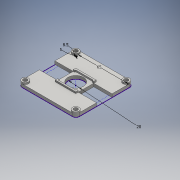
# Autodesk Inventor part: 20mm glass cuvette holder
Saved by Autodesk Inventor 2016 SP1 (Build 200210100, 210)
## iProperties
Created: 2015-08-25
Part Number: 20mm glass cuvette holder
Material: Generic
Document SubType Name: Modeling
Designer: kthorn
Density: 1 g/cm^3
Appearance: Default
Author: kthorn
Autodesk Inventor part; units mm, degrees
ref_plane "YZ Plane" through (0, 0, 0) normal (1, 0, 0) x (0, 1, 0)
ref_plane "XZ Plane" through (0, 0, 0) normal (0, 1, 0) x (-1, 0, 0)
ref_plane "XY Plane" through (0, 0, 0) normal (0, 0, 1) x (1, 0, 0)
sketch "Sketch1" plane through (0, 0, 0) normal (0, 0, 1) x (1, 0, 0)
  line L0 (-32.5, 32.5) -> (32.5, 32.5) construction
  line L1 (32.5, 32.5) -> (32.5, -32.5) construction
  line L2 (32.5, -32.5) -> (-32.5, -32.5) construction
  line L3 (-32.5, -32.5) -> (-32.5, 32.5) construction
  circle A0 centre (-32.5, 32.5) radius 2.5
  circle A1 centre (32.5, 32.5) radius 2.5
  circle A2 centre (-32.5, -32.5) radius 2.5
  circle A3 centre (32.5, -32.5) radius 2.5
  line L4 (-32.5, 32.5) -> (32.5, -32.5) construction
  circle A4 centre (0, 0) radius 10
  circle A5 centre (-32.5, 32.5) radius 4.25
  circle A6 centre (32.5, 32.5) radius 4.25
  circle A7 centre (-32.5, -32.5) radius 4.25
  circle A8 centre (32.5, -32.5) radius 4.25
  line L5 (-32.5, 36.75) -> (32.5, 36.75)
  line L6 (32.5, -36.75) -> (-32.5, -36.75)
  line L7 (-36.75, 32.5) -> (-36.75, -32.5)
  line L8 (36.75, 32.5) -> (36.75, -32.5)
  dimension "d1" = 65
  dimension "d2" = 5
  dimension "d4" = 20
  dimension "d16" = 8.5
  constraints: 18 end point, 9 centre point, 9 coincident, 8 point on circle, 7 tangent, 6 equal radius, 2 horizontal, 2 parallel, 2 perpendicular, 1 midpoint
  measures "d1" distance of L0.start L0.end
  measures "d2" diameter of A0
  measures "d4" diameter of A4
  measures "d16" diameter of A5
extrude "Extrusion1" add sketch "Sketch1" along normal blind 4
sketch "Sketch2" plane through (0, 0, 4) normal (0, 0, 1) x (1, 0, 0)
  line L0 (-11.2, 11.2) -> (11.2, 11.2)
  line L1 (11.2, -11.2) -> (-11.2, -11.2)
  line L2 (0, 11.2) -> (0, 36.75) construction
  line L3 (0, -11.2) -> (0, -36.75) construction
  line L4 (-13.2, 13.2) -> (13.2, 13.2)
  line L5 (13.2, -13.2) -> (-13.2, -13.2)
  line L6 (11.2, 11.2) -> (13.2, 13.2) construction
  line L7 (-11.2, 11.2) -> (-13.2, 13.2) construction
  line L8 (-13.2, -13.2) -> (-11.2, -11.2) construction
  line L9 (11.2, -11.2) -> (13.2, -13.2) construction
  circle A0 centre (0, 0) radius 10 projected
  circle A1 centre (-32.5, -32.5) radius 2.5 projected
  circle A2 centre (32.5, -32.5) radius 2.5 projected
  circle A3 centre (32.5, 32.5) radius 2.5 projected
  circle A4 centre (-32.5, 32.5) radius 2.5 projected
  arc A5 (32.5, -36.75) -> (36.75, -32.5) centre (32.5, -32.5) ccw projected
  line L10 (36.75, -32.5) -> (36.75, 32.5) projected
  arc A6 (36.75, 32.5) -> (32.5, 36.75) centre (32.5, 32.5) ccw projected
  line L11 (32.5, 36.75) -> (-32.5, 36.75) projected
  arc A7 (-32.5, 36.75) -> (-36.75, 32.5) centre (-32.5, 32.5) ccw projected
  line L12 (-36.75, 32.5) -> (-36.75, -32.5) projected
  arc A8 (-36.75, -32.5) -> (-32.5, -36.75) centre (-32.5, -32.5) ccw projected
  line L13 (-32.5, -36.75) -> (32.5, -36.75) projected
  line L14 (-32.5, -36.75) -> (32.5, -36.75) projected
  line L15 (36.75, -32.5) -> (36.75, 32.5) projected
  line L16 (32.5, 36.75) -> (-32.5, 36.75) projected
  line L17 (-13.2, 10) -> (-11.2, 10)
  line L18 (-13.2, -10) -> (-11.2, -10)
  line L19 (-13.2, -13.2) -> (-13.2, -10)
  line L20 (-13.2, 10) -> (-13.2, 13.2)
  line L21 (-11.2, -11.2) -> (-11.2, -10)
  line L22 (-11.2, 10) -> (-11.2, 11.2)
  line L23 (11.2, 10) -> (13.2, 10)
  line L24 (11.2, -10) -> (13.2, -10)
  line L25 (11.2, 11.2) -> (11.2, 10)
  line L26 (11.2, -10) -> (11.2, -11.2)
  line L27 (13.2, 13.2) -> (13.2, 10)
  line L28 (13.2, -10) -> (13.2, -13.2)
  line L29 (-11.2, 11.2) -> (0, 0) construction
  line L30 (0, 0) -> (-11.2, -11.2) construction
  line L31 (0, 0) -> (11.2, 11.2) construction
  line L32 (0, 0) -> (11.2, -11.2) construction
  dimension "d7" = 22.4
  dimension "d24" = 2
  dimension "d31" = 2
  dimension "d34" = 20
  constraints: 52 end point, 14 perpendicular, 12 equal length, 10 parallel, 4 midpoint, 2 horizontal, 2 point on line, 1 vertical
  measures "d7" distance of L0.start L0.end
  measures "d24" distance of L17.start L17.end
  measures "d31" distance between parallel lines of L0 L4
  measures "d34" distance from line of L18.end L17
extrude "Extrusion2" add sketch "Sketch2" along normal blind 2 contours L22 L17 L20 L4 L27 L23 L25 L0 | L26 L24 L28 L5 L19 L18 L21 L1
extrude "Extrusion4" add sketch "Sketch1" along normal blind 6 contours A5 | A6 | A7 | A8
sketch "Sketch4" plane through (0, 0, 4) normal (0, 0, 1) x (1, 0, 0)
  line L0 (13.2, 13.2) -> (13.2, 10) projected
  line L1 (-13.2, 13.2) -> (13.2, 13.2) projected
  arc A0 (36.75, -32.5) -> (32.5, -36.75) centre (32.5, -32.5) ccw projected
  line L2 (36.75, -32.5) -> (36.75, 32.5) projected
  arc A1 (32.5, 36.75) -> (36.75, 32.5) centre (32.5, 32.5) ccw projected
  line L3 (32.5, 36.75) -> (-32.5, 36.75) projected
  arc A2 (-36.75, 32.5) -> (-32.5, 36.75) centre (-32.5, 32.5) ccw projected
  line L4 (-36.75, 32.5) -> (-36.75, -32.5) projected
  arc A3 (-32.5, -36.75) -> (-36.75, -32.5) centre (-32.5, -32.5) ccw projected
  line L5 (-32.5, -36.75) -> (32.5, -36.75) projected
  line L6 (-13.2, 10) -> (-13.2, -10)
  line L7 (-13.2, -10) -> (-36.75, -10)
  line L8 (-36.75, -10) -> (-36.75, 10)
  line L9 (-36.75, 10) -> (-13.2, 10)
  line L10 (32.5, 36.75) -> (-32.5, 36.75) construction
  line L11 (0, 36.75) -> (0, -36.75) construction
  line L12 (13.2, 10) -> (13.2, -10)
  line L13 (13.2, -10) -> (36.75, -10)
  line L14 (36.75, -10) -> (36.75, 10)
  line L15 (36.75, 10) -> (13.2, 10)
  line L16 (-11.2, 11.2) -> (-11.2, 10) projected
  line L17 (-11.2, 10) -> (-13.2, 10) projected
  line L18 (-13.2, 10) -> (-13.2, 13.2) projected
  line L19 (13.2, 10) -> (11.2, 10) projected
  line L20 (11.2, 10) -> (11.2, 11.2) projected
  line L21 (11.2, 11.2) -> (-11.2, 11.2) projected
  line L22 (-11.2, 11.2) -> (11.2, 11.2) projected
  line L23 (11.2, 11.2) -> (11.2, 10) projected
  line L24 (11.2, 10) -> (13.2, 10) projected
  line L25 (13.2, 10) -> (13.2, 13.2) projected
  line L26 (13.2, 13.2) -> (-13.2, 13.2) projected
  line L27 (-13.2, 13.2) -> (-13.2, 10) projected
  line L28 (-13.2, 10) -> (-11.2, 10) projected
  line L29 (-11.2, 10) -> (-11.2, 11.2) projected
  line L30 (-11.2, -11.2) -> (-11.2, -10) projected
  line L31 (-13.2, -10) -> (-13.2, -13.2) projected
  line L32 (-13.2, 13.2) -> (-13.2, 10) projected
  circle A4 centre (0, 0) radius 10 projected
  line L33 (-11.2, -11.2) -> (11.2, -11.2) projected
  line L34 (11.2, -11.2) -> (11.2, -10) projected
  line L35 (11.2, -10) -> (13.2, -10) projected
  line L36 (13.2, -10) -> (13.2, -13.2) projected
  line L37 (13.2, -13.2) -> (-13.2, -13.2) projected
  line L38 (-13.2, -13.2) -> (-13.2, -10) projected
  line L39 (-13.2, -10) -> (-11.2, -10) projected
  line L40 (-11.2, -10) -> (-11.2, -11.2) projected
  point P0 (-36.75, 0)
  point P1 (36.75, 0)
  dimension "d20" = 20
  constraints: 18 end point, 5 symmetric about line, 4 midpoint, 2 parallel, 1 perpendicular, 1 point on line
  measures "d20" distance between parallel lines of L7 L9
extrude "Extrusion5" cut sketch "Sketch4" against normal through all contours L15 L2 L13 L12 | L6 L7 L4 L9
body "Solid1"
